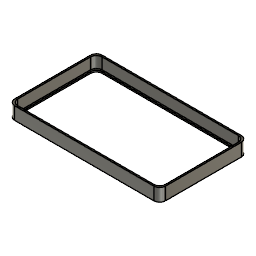
Screen Holder (Autodesk Fusion 360 design; units mm, degrees)
Autodesk Fusion 360 part; units mm, degrees
sketch "Sketch1" plane through (0, 0, 0) normal (0, 0, 1) x (1, 0, 0)
  line L0 (-96.875, 55.375) -> (96.875, 55.375)
  line L1 (96.875, 55.375) -> (96.875, -55.375)
  line L2 (96.875, -55.375) -> (-96.875, -55.375)
  line L3 (-96.875, -55.375) -> (-96.875, 55.375)
  line L4 (-98.875, 57.375) -> (98.875, 57.375)
  line L5 (98.875, 57.375) -> (98.875, -57.375)
  line L6 (98.875, -57.375) -> (-98.875, -57.375)
  line L7 (-98.875, -57.375) -> (-98.875, 57.375)
  point P0 (0, 55.375)
  point P1 (-96.875, 0)
  point P2 (0, 57.375)
  point P3 (98.875, 0)
  dimension "d1" = 193.75
  dimension "d2" = 110.75
  dimension "d3" = 2
  dimension "d4" = 2
  constraint horizontal L0
  constraint vertical L1
  constraint horizontal L2
  constraint vertical L3
  constraint midpoint L0 P0
  constraint midpoint L3 P1
  constraint horizontal origin P1
  constraint vertical origin P0
  constraint horizontal L4
  constraint vertical L5
  constraint horizontal L6
  constraint vertical L7
  constraint midpoint L4 P2
  constraint midpoint L5 P3
  constraint vertical origin P2
  constraint horizontal origin P3
  measures "d1" distance of L0.start L0.end
  measures "d2" distance of L0.end L1.end
  measures "d3" distance of L0 L4
  measures "d4" distance of L1 L5
extrude "Extrude1" add sketch "Sketch1" along normal blind 14.8
sketch "Sketch2" plane through (0, 0, 0) normal (0, 0, -1) x (1, 0, 0)
  line L0 (-96.875, 55.375) -> (96.875, 55.375)
  line L1 (96.875, 55.375) -> (96.875, -55.375)
  line L2 (96.875, -55.375) -> (-96.875, -55.375)
  line L3 (-96.875, -55.375) -> (-96.875, 55.375)
  line L4 (98.875, 57.375) -> (-98.875, 57.375)
  line L5 (-98.875, 57.375) -> (-98.875, -57.375)
  line L6 (-98.875, -57.375) -> (98.875, -57.375)
  line L7 (98.875, -57.375) -> (98.875, 57.375)
  line L8 (-98.875, 57.375) -> (98.875, 57.375)
  line L9 (98.875, 57.375) -> (98.875, -57.375)
  line L10 (98.875, -57.375) -> (-98.875, -57.375)
  line L11 (-98.875, -57.375) -> (-98.875, 57.375)
  line L12 (-94.875, 53.375) -> (94.875, 53.375)
  line L13 (94.875, 53.375) -> (94.875, -53.375)
  line L14 (94.875, -53.375) -> (-94.875, -53.375)
  line L15 (-94.875, -53.375) -> (-94.875, 53.375)
  point P0 (0, 53.375)
  point P1 (94.875, 0)
  dimension "d15" = 2
  dimension "d16" = 2
  constraint horizontal L8
  constraint vertical L9
  constraint horizontal L10
  constraint vertical L11
  constraint coincident L6.end L7.start
  constraint coincident L4.end L5.start
  constraint horizontal L12
  constraint vertical L13
  constraint horizontal L14
  constraint vertical L15
  constraint midpoint L12 P0
  constraint midpoint L13 P1
  constraint vertical origin P0
  constraint horizontal origin P1
  measures "d15" distance of L1 L13
  measures "d16" distance of L2 L14
extrude "Extrude2" add sketch "Sketch2" along normal blind 2 contours L0 L1 L2 L3 | L4 L5 L6 L7 L8 L9 L10 L11
fillet "Fillet1" radius 7.5 12 edges at (-94.875, -53.375, -1) (-94.875, 53.375, -1) (94.875, 53.375, -1) (94.875, -53.375, -1) (-98.875, 57.375, 6.4) (-98.875, -57.375, 6.4) (98.875, 57.375, 6.4) (98.875, -57.375, 6.4) (96.875, 55.375, 7.4) (96.875, -55.375, 7.4) (-96.875, -55.375, 7.4) (-96.875, 55.375, 7.4)
equation "d4 = d3"
equation "d5 = 2 mm + 4.8 mm + 8 mm"
equation "d16 = d15"
